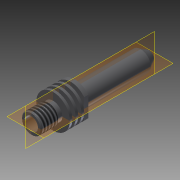
# Autodesk Inventor part: D-039
Saved by Autodesk Inventor 2015 (Build 190159000, 159)
## iProperties
Company: MARCHA TECHNOLOGY
Created: 2014-03-07
Part Number: D-039
Document SubType Name: Modeling
Designer: O.Martin
Density: 1 g/cm^3
Project: WITBOXprinter_K01
Description: HOT END TORNILLO
Stock Number: 28655
Mass: 0.769904 g
Surface Area: 15.7397 cm^2
Volume: 0.769904 cm^3
Material: Generic
Appearance: Gray
Author: O.Martin
Autodesk Inventor part; units mm, degrees
ref_plane "XZ Plane" through (0, 0, 0) normal (0, 1, 0) x (-1, 0, 0)
sketch "Boceto1" plane through (0, 0, 0) normal (0, 0, 1) x (1, 0, 0)
  line L0 (0, 0) -> (0, 35)
  line L1 (0, 35) -> (-3, 35)
  line L2 (-3, 35) -> (-3, 13)
  line L3 (-3, 5) -> (-3, 0)
  line L4 (-3, 0) -> (0, 0)
  line L5 (-2, 31) -> (-2, 0)
  line L6 (-5, 6.5) -> (-5, 13)
  line L7 (-3, 13) -> (-5, 13)
  line L8 (-3, 5) -> (-2.75, 5.25)
  line L9 (-2.75, 5.25) -> (-2.75, 6.5)
  line L10 (-2.75, 6.5) -> (-5, 6.5)
  line L11 (-5, 7.25) -> (-3, 7.25)
  line L12 (-3, 7.25) -> (-3, 8.25)
  line L13 (-3, 8.25) -> (-5, 8.25)
  line L14 (-5, 8.25) -> (-5, 7.25)
  line L15 (-5, 9) -> (-3, 9)
  line L16 (-3, 9) -> (-3, 10)
  line L17 (-3, 10) -> (-5, 10)
  line L18 (-5, 10) -> (-5, 9)
  line L19 (-5, 10.75) -> (-3, 10.75)
  line L20 (-3, 10.75) -> (-3, 11.75)
  line L21 (-3, 11.75) -> (-5, 11.75)
  line L22 (-5, 11.75) -> (-5, 10.75)
  line L23 (-3, 16.2679) -> (-2, 18)
  line L24 (-2, 18) -> (-3, 19.7321)
  line L25 (-2, 31) -> (-1, 31.5774)
  line L26 (-1, 31.5774) -> (-1, 34)
  line L27 (-1, 34) -> (-1.5774, 35)
  line L28 (-1, 0) -> (-1, 6)
  line L29 (-1, 6) -> (-2, 6)
  line L30 (-2, 31) -> (-2, 34)
  line L31 (-3, 32.25) -> (-1.9896, 34)
  line L32 (-2, 34) -> (-1.9896, 34)
  dimension "d0" = 6
  dimension "d3" = 6
  dimension "d6" = 4
  dimension "d32" = 10
  dimension "d33" = 13
  dimension "d42" = 5.5
  dimension "d43" = 5
  dimension "d44" = 45
  dimension "d45" = 1.5
  dimension "d46" = 2
  dimension "d47" = 2
  dimension "d48" = 1
  dimension "d50" = 0.75
  dimension "d51" = 0.75
  dimension "d52" = 0.75
  dimension "d55" = 1
  dimension "d56" = 5
  dimension "d57" = 60
  dimension "d58" = 2
  dimension "d60" = 1
  dimension "d98" = 2
  dimension "d99" = 6
  dimension "d103" = 30
  dimension "d112" = 22
  dimension "d113" = 2.75
  dimension "d114" = 31
  constraints: 66 end point, 13 perpendicular, 10 parallel, 10 point on line, 4 equal length, 3 horizontal, 1 collinear, 1 vertical
  measures "d0" diameter of L3 L0
  measures "d3" diameter of L2 L0
  measures "d6" diameter of L5 L0
  measures "d32" diameter of L6 L0
  measures "d33" distance between parallel lines of L7 L4
  measures "d42" diameter of L9 L0
  measures "d43" distance of L3.start L3.end
  measures "d44" angle of L9 L8
  measures "d45" distance from line of L10 L3.start
  measures "d46" distance of L11.start L11.end
  measures "d47" distance of L15.start L15.end
  measures "d48" distance between parallel lines of L13 L11
  measures "d50" distance between parallel lines of L10 L11
  measures "d51" distance between parallel lines of L13 L15
  measures "d52" distance between parallel lines of L17 L19
  measures "d55" distance from line of L2 L23.end
  measures "d56" distance from line of L7 L23.end
  measures "d57" angle of L5 L25
  measures "d58" diameter of L26 L0
  measures "d60" vertical distance of L26.end L27.end
  measures "d98" diameter of L28 L0
  measures "d99" distance of L28.start L28.end
  measures "d103" angle of L2 L31
  measures "d112" distance between parallel lines of L1 L7
  measures "d113" distance from line of L31.start L1
  measures "d114" distance from line of L4 L5.start
revolve "Revolución1" add sketch "Boceto1" angle 360 about axis through (0, 0, 0) along (0, 1, 0) contours L30 L32 L31 | L27 L26 L25 L30 L31 L2 L1 | L4 L3 L8 L9 L10 L6 L11 L12 L13 L15 L16 L17 L19 L20 L21 L7 L2 L23 L5 | L31 L30 L5 L24 L2 | L23 L2 L24
thread "Rosca1" size "M6x1" class "6g" standard "ANSI Metric M Profile" full length
chamfer "Chaflán1" distance 0.25 angle 45 1 edges at (3, 0, 0)
chamfer "Chaflán4" distance 2.4 angle 30 1 edges at (3, 35, 0) measured on face at (3, 34.5, 0)
sketch "Boceto7" plane through (0, 13, 0) normal (0, 1, 0) x (1, 0, 0)
  circle A0 centre (0, 0) radius 5 projected
  line L0 (-4, 3) -> (-4, -3)
  line L1 (4, 3) -> (4, -3)
  circle A1 centre (0, 0) radius 5 projected
  dimension "d109" = 8
  constraints: 4 end point, 4 point on circle, 2 parallel, 1 vertical, 2 other
  measures "d109" distance between parallel lines of L1 L0
extrude "Extrusión5" cut sketch "Boceto7" against normal blind 2 contours A0 L1 | L0 A0
sketch "Boceto3" plane through (0, 0, 0) normal (0, 0, 1) x (1, 0, 0)
  line L0 (2.995, 37) -> (-2.995, 37) projected
  circle A0 centre (-6, 39.5) radius 6.25 construction
  circle A1 centre (5.2404, 39.9651) radius 5 construction
  circle A2 centre (-6, 39.5) radius 5.45
  circle A3 centre (5.2404, 39.9651) radius 5.2
  dimension "d72" = 0.2
  dimension "d76" = 10.9
  constraints: 2 centre point, 2 coincident
  measures "d72" radial gap between concentric circles of A3 A1
  measures "d76" diameter of A2
sketch "Boceto6" plane through (0, 24, 0) normal (0, 1, 0) x (1, 0, 0)
  circle A0 centre (0, 0) radius 3.05 projected
  line L0 (1.3191, -2.75) -> (-1.3191, -2.75)
  dimension "d91" = 0.3
  constraints: 2 end point, 2 point on circle, 1 horizontal
  measures "d91" distance edge to line of A0 L0
sketch "Boceto5" plane through (-6, 0, 0) normal (1, 0, 0) x (0, 1, 0)
  line L0 (45.75, 4) -> (33.25, 4) construction
  line L1 (45.75, 4) -> (45.75, 2) construction
  line L2 (45.7644, -2) -> (45.7644, -4) construction
  arc A0 (45.75, 2) -> (45.7644, -2) centre (47.2393, 0.0053) ccw construction
  line L3 (39.5, 4) -> (39.5, -4)
  line L4 (45.7644, -4) -> (39.5, -4) construction
  arc A1 (45.95, 1.8971) -> (45.9644, -1.8961) centre (47.2393, 0.0053) ccw
  line L5 (45.9644, -4.2) -> (42.2056, -4.2)
  line L6 (45.9644, 4.4) -> (42.2056, 4.4)
  line L7 (42.2056, 4.4) -> (42.2056, -4.2)
  line L8 (45.9644, 4.4) -> (45.9644, -4.2)
  dimension "d82" = 4
  dimension "d83" = 2
  dimension "d84" = 10.5
  dimension "d85" = 0.2
  dimension "d87" = 2.2893
  dimension "d89" = 3.7932
  constraints: 16 end point, 5 parallel, 4 point on circle, 3 perpendicular, 2 centre point, 1 midpoint
  measures "d82" vertical distance of L2.start L1.end
  measures "d83" distance of L0.start L1.end
  measures "d85" radial gap between concentric circles of A1 A0
  measures "d87" radius of A1
  measures "d89" vertical distance of A1.start A1.end
equation "\"d51\" = d50"
equation "\"d52\" = d51"
body "Solid1"
